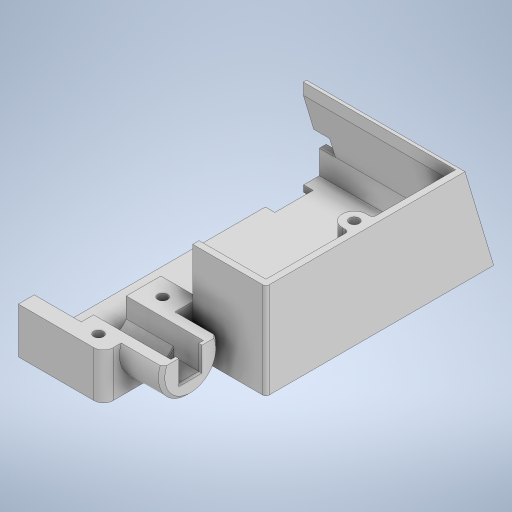
# Autodesk Inventor part: Tělo
Saved by Autodesk Inventor 2024 (Build 280153000, 153)
## iProperties
Created: 2023-04-15
Part Number: Tělo
Material: Všeobecné
Document SubType Name: Modeling
Designer: 42060
Density: 1 g/cm^3
Appearance: Výchozí
Author: 42060
Autodesk Inventor part; units mm, degrees
ref_plane "YZ Plane" through (0, 0, 0) normal (1, 0, 0) x (0, 1, 0)
ref_plane "XZ Plane" through (0, 0, 0) normal (0, 1, 0) x (-1, 0, 0)
ref_plane "XY Plane" through (0, 0, 0) normal (0, 0, 1) x (1, 0, 0)
sketch "Základ" plane through (0, 0, 0) normal (0, 0, 1) x (1, 0, 0)
  line L0 (0, 0) -> (49.75, 0)
  line L1 (49.75, 0) -> (49.75, -71.5)
  line L2 (49.75, -71.5) -> (26.75, -71.5)
  line L3 (26.75, -99.5) -> (0, -99.5)
  line L4 (0, -99.5) -> (0, 0)
  line L5 (0, -10) -> (47.75, -10)
  line L6 (47.75, -10) -> (47.75, -69.5)
  line L7 (47.75, -69.5) -> (14.75, -69.5)
  line L8 (14.75, -69.5) -> (14.75, -94.5)
  line L9 (14.75, -94.5) -> (0, -94.5)
  line L10 (26.75, -71.5) -> (26.75, -80.375)
  line L11 (26.75, -80.375) -> (26.75, -90.625)
  line L12 (26.75, -90.625) -> (26.75, -99.5)
  line L13 (26.75, -90.625) -> (14.75, -90.625)
  line L14 (26.75, -80.375) -> (14.75, -80.375)
  line L15 (26.75, -71.5) -> (26.75, -69.5)
  dimension "d0" = 49.75
  dimension "d1" = 99.5
  dimension "d3" = 2
  dimension "d5" = 28
  dimension "d14" = 10.25
  dimension "d15" = 12
  dimension "d16" = 5
  dimension "d17" = 23
  dimension "d18" = 2
  dimension "d19" = 10
  constraints: 32 end point, 8 perpendicular, 6 point on line, 3 horizontal, 2 collinear, 1 parallel, 1 vertical
  measures "d0" distance of L0.start L0.end
  measures "d1" distance between parallel lines of L3 L0
  measures "d3" distance between parallel lines of L1 L6
  measures "d5" distance of L2.end L3.start
  measures "d14" distance of L10.end L11.end
  measures "d15" distance between parallel lines of L8 L10
  measures "d16" distance between parallel lines of L9 L3
  measures "d17" distance between parallel lines of L1 L12
  measures "d18" distance between parallel lines of L2 L7
  measures "d19" distance between parallel lines of L0 L5
extrude "Podlaha" add sketch "Základ" along normal blind 2 contours L5 L6 L7 L8 L9 L4
extrude "Stěny" add sketch "Základ" along normal blind 30 contours L0 L1 L2 L15 L7 L6 L5 L4
extrude "Zadní stěny" add sketch "Základ" along normal blind 15 contours L9 L8 L13 L12 L3 L4 | L10 L14 L8 L7 L15
extrude "Stěna pod motorem" add sketch "Základ" along normal blind 5.25 contours L11 L13 L8 L14
sketch "Náčrt2" plane through (49.75, -71.5, 0) normal (1, 0, 0) x (0, 0, -1)
  line L0 (-2, 61.5) -> (-30, 61.5) projected
  line L1 (-2, 61.5) -> (-30, 61.5) projected
  line L2 (-30, 0) -> (-30, 71.5) projected
  line L3 (0, 71.5) -> (-30, 71.5) projected
  line L4 (0, 71.5) -> (0, 0) projected
  line L5 (-30, 62.5) -> (-10, 68.5)
  line L6 (-10, 68.5) -> (0, 71.5)
  dimension "d28" = 1
  dimension "d30" = 20
  constraints: 4 end point, 1 collinear, 1 point on line
  measures "d28" distance from line of L5.start L0
  measures "d30" horizontal distance of L5.end L5.start
extrude "Rampa" cut sketch "Náčrt2" against normal through all
sketch "Náčrt3" plane through (0, -10, 2) normal (-1, 0, 0) x (0, 0, 1)
  line L0 (0, 0) -> (28, 0) projected
  line L1 (0, 0) -> (28, 0) projected
  line L2 (24.3731, 0) -> (7.5, 5.0619)
  line L3 (7.5, 5.0619) -> (0, 5.0619)
  line L4 (0, 5.0619) -> (0, 0)
  line L5 (28, 1) -> (-2, 10) projected
  point P0 (-2, 10)
  point P1 (2, 7)
  point P2 (24.3731, 0)
  dimension "d34" = 7.5
  dimension "d37" = 2
  constraints: 6 end point, 1 horizontal, 1 perpendicular, 1 point on line, 2 other
  measures "d34" distance of L2.end L3.end
extrude "Přední rampa" cut sketch "Náčrt3" against normal up to surface (47.75 mm away)
sketch "Držák motoru" plane through (14.75, -94.5, 2) normal (-1, 0, 0) x (0, 0, 1)
  line L0 (3.25, 14.125) -> (13, 14.125) projected
  line L1 (3.25, 14.125) -> (3.25, 3.875) projected
  line L2 (3.25, 3.875) -> (13, 3.875) projected
  line L3 (6.13, 14.125) -> (12.37, 14.125)
  line L4 (12.37, 3.875) -> (6.13, 3.875)
  line L5 (3.25, 3.875) -> (13, 3.875) projected
  arc A0 (12.37, 3.875) -> (12.37, 14.125) centre (9.25, 9) ccw
  arc A1 (6.13, 14.125) -> (6.13, 3.875) centre (9.25, 9) ccw
  line L6 (15.25, 14.125) -> (15.25, 3.875) construction
  circle A2 centre (9.25, 9) radius 9
  line L7 (9.25, 18) -> (0, 18)
  line L8 (0, 0) -> (0, 89.5619) projected
  line L9 (0, 0) -> (13, 0) projected
  line L10 (13, -5) -> (13, 3.875) projected
  line L11 (0, 0) -> (13, 0) projected
  line L12 (0, 0) -> (13, 0) projected
  line L13 (12.37, 14.125) -> (12.37, 17.4419)
  line L14 (12.37, 3.875) -> (12.37, 0.5581)
  line L15 (12.37, 0.5581) -> (12.37, 0)
  line L16 (12.37, 17.4419) -> (12.37, 18)
  line L17 (12.37, 18) -> (9.25, 18)
  point P0 (-2, 94.5)
  point P1 (15.25, 9)
  point P2 (15.25, 9)
  point P3 (3.25, 9)
  point P4 (3.25, 9)
  point P5 (6.13, 3.875)
  point P6 (9.25, 0)
  point P7 (16.7333, 14)
  point P8 (16.7333, 4)
  point P9 (12.37, 0)
  dimension "d38" = 6
  dimension "d39" = 6
  dimension "d41" = 3
  dimension "d48" = 12
  constraints: 18 end point, 9 point on circle, 7 point on line, 4 tangent, 3 centre point, 3 coincident, 3 vertical, 2 horizontal alignment, 2 midpoint, 1 horizontal, 1 perpendicular
  measures "d38" radius of A0
  measures "d39" radius of A1
  measures "d41" radial gap between concentric circles of A2 A0
  measures "d48" distance between parallel lines of L1 L6
sketch "Náčrt10" plane through (14.75, -99.5, 0) normal (1, 0, 0) x (0, 0, -1)
  line L0 (-5.25, 8.875) -> (-15, 8.875) construction
  line L1 (-5.25, 8.875) -> (-17.25, 8.875) construction
  line L2 (-17.25, 8.875) -> (-17.25, 19.125) construction
  line L3 (-17.25, 19.125) -> (-5.25, 19.125) construction
  line L4 (-5.25, 19.125) -> (-5.25, 8.875) construction
  line L5 (-14.37, 8.875) -> (-8.13, 8.875)
  arc A0 (-8.13, 8.875) -> (-8.13, 19.125) centre (-11.25, 14) ccw
  line L6 (-14.37, 19.125) -> (-8.13, 19.125)
  arc A1 (-14.37, 5.5581) -> (-14.37, 22.4419) centre (-11.25, 14) ccw
  line L7 (-14.37, 8.875) -> (-14.37, 5.5581)
  line L8 (-14.37, 19.125) -> (-14.37, 22.4419)
  point P0 (0, 99.5)
  point P1 (-11.25, 19.125)
  point P2 (-11.25, 19.125)
  point P3 (-11.25, 8.875)
  point P4 (-11.25, 8.875)
  dimension "d79" = 12
  dimension "d80" = 6
  dimension "d81" = 18
  constraints: 16 end point, 5 point on line, 4 midpoint, 4 point on circle, 3 coincident, 2 centre point, 2 parallel, 2 perpendicular, 2 vertical alignment, 1 collinear, 1 horizontal, 1 horizontal alignment, 1 tangent
  measures "d79" distance between parallel lines of L4 L2
  measures "d80" radius of A0
  measures "d81" diameter of A1
extrude "Držák motoru (kulaté)" add sketch "Náčrt10" along normal blind 15
sketch "Náčrt11" plane through (29.75, -99.5, 0) normal (1, 0, 0) x (0, 0, -1)
  arc A0 (-8.13, 8.875) -> (-8.13, 19.125) centre (-11.25, 14) ccw projected
  circle A1 centre (-11.25, 14) radius 9
  line L0 (-17.25, 8.875) -> (-5.25, 8.875)
  line L1 (-5.25, 8.875) -> (-5.25, 19.125)
  line L2 (-5.25, 19.125) -> (-17.25, 19.125)
  line L3 (-17.25, 19.125) -> (-17.25, 8.875)
  line L4 (-17.25, 8.875) -> (-5.25, 19.125) construction
  line L5 (-5.25, 8.875) -> (-17.25, 19.125) construction
  line L6 (-14.37, 8.875) -> (-14.37, 5.5581) projected
  line L7 (-14.37, 22.4419) -> (-14.37, 19.125) projected
  point P0 (0, 99.5)
  dimension "d84" = 18
  constraints: 12 end point, 2 midpoint, 2 parallel, 1 centre point, 1 coincident, 1 horizontal, 1 horizontal alignment, 1 perpendicular, 1 tangent
  measures "d84" diameter of A1
extrude "Držák motoru (hranaté)" add sketch "Náčrt11" along normal blind 9.25 contours L0 L1 L2 L7 A1 L6
sketch "Spodní senzory" plane through (0, 0, 2) normal (0, 0, 1) x (1, 0, 0)
  line L0 (0, -4.9381) -> (47.75, -4.9381) projected
  line L1 (0, -94.5) -> (0, -4.9381) projected
  line L2 (0, -94.5) -> (14.75, -94.5) projected
  line L3 (14.75, -94.5) -> (14.75, -69.5) projected
  line L4 (14.75, -69.5) -> (47.75, -69.5) projected
  line L5 (47.75, -69.5) -> (47.75, -4.9381) projected
  line L6 (0, -24.4381) -> (5.5, -24.4381)
  line L7 (0, -21.9381) -> (3, -21.9381)
  line L8 (3, -21.9381) -> (3, -9.9381)
  line L9 (3, -9.9381) -> (0, -9.9381)
  line L10 (0, -7.4381) -> (5.5, -7.4381)
  line L11 (5.5, -7.4381) -> (5.5, -24.4381)
  line L12 (47.75, -22.8381) -> (36.75, -22.8381)
  line L13 (36.75, -22.8381) -> (36.75, -4.9381)
  line L14 (45.25, -20.3381) -> (39.25, -20.3381)
  line L15 (39.25, -20.3381) -> (39.25, -8.3381)
  line L16 (39.25, -8.3381) -> (45.25, -8.3381)
  line L17 (45.25, -8.3381) -> (45.25, -20.3381)
  point P0 (0, 0)
  dimension "d155" = 3
  dimension "d157" = 12
  dimension "d159" = 2.5
  dimension "d163" = 5
  dimension "d170" = 2.5
  dimension "d171" = 2.5
  dimension "d174" = 2.5
  dimension "d175" = 2.5
  dimension "d176" = 2.5
  dimension "d177" = 12
  dimension "d178" = 6
  dimension "d179" = 3.4
  constraints: 24 end point, 6 point on line, 5 perpendicular, 4 horizontal, 2 parallel, 1 vertical
  measures "d155" distance of L7.start L7.end
  measures "d157" distance of L7.end L8.end
  measures "d159" distance between parallel lines of L7 L6
  measures "d163" distance between parallel lines of L0 L9
  measures "d170" distance between parallel lines of L10 L9
  measures "d171" distance between parallel lines of L8 L11
  measures "d174" distance between parallel lines of L13 L15
  measures "d175" distance between parallel lines of L5 L17
  measures "d176" distance between parallel lines of L14 L12
  measures "d177" distance of L14.end L15.end
  measures "d178" distance of L14.start L14.end
  measures "d179" distance between parallel lines of L0 L16
extrude "Spodní senzory (díra)" cut sketch "Spodní senzory" against normal through all contours L9 L8 L7 L1 | L14 L15 L16 L17
extrude "Spodní senzory zvýšení" add sketch "Spodní senzory" along normal blind 10.5 contours L0 L5 L12 L13
sketch "Náčrt12" plane through (0, 0, 15) normal (0, 0, 1) x (1, 0, 0)
  line L0 (26.75, -80.375) -> (26.75, -71.5) projected
  line L1 (26.75, -69.5) -> (26.75, -71.5) projected
  line L2 (26.75, -69.5) -> (14.75, -69.5) projected
  line L3 (14.75, -69.5) -> (14.75, -80.375) projected
  line L4 (14.75, -80.375) -> (26.75, -80.375) projected
  line L5 (26.75, -99.5) -> (26.75, -90.625) projected
  line L6 (26.75, -90.625) -> (14.75, -90.625) projected
  line L7 (14.75, -90.625) -> (14.75, -94.5) projected
  line L8 (14.75, -94.5) -> (0, -94.5) projected
  line L9 (0, -94.5) -> (0, -99.5) projected
  line L10 (0, -99.5) -> (26.75, -99.5) projected
  point P0 (0, 0)
extrude "Vyrovnání držáku motoru" cut sketch "Náčrt12" against normal up to surface (0.63 mm away)
sketch "Náčrt13" plane through (14.75, -80.375, 14.37) normal (0, 0, 1) x (1, 0, 0)
  line L0 (0, 0) -> (0, 10.875) projected
  line L1 (0, 10.875) -> (12, 10.875) projected
  line L2 (0, -14.125) -> (0, -10.25) projected
  line L3 (0, -10.25) -> (24.25, -10.25) projected
  point P0 (-14.75, 80.375)
  point P1 (6, 5.4375)
  point P2 (6, -14.6875)
  dimension "d89" = 6
  dimension "d90" = 5.4375
  dimension "d91" = 6
  dimension "d92" = 4.4375
  measures "d89" distance from line of L0 point (6, 5.438)
  measures "d90" distance from line of L1 point (6, 5.438)
  measures "d91" distance from line of L2 point (6, -14.687)
  measures "d92" distance from line of L3 point (6, -14.687)
hole "Díry pro objímku motoru" at (20.75, -95.0625, 14.37) at (20.75, -74.9375, 14.37) direction (0, 0, -1) diameter 3 depth 6
fillet "Zaoblení stěny motoru" radius 3 1 edges at (26.75, -99.5, 7.185)
fillet "Zaoblení stěny" radius 1 1 edges at (49.75, -71.5, 15)
sketch "Náčrt14" plane through (39, -99.5, 0) normal (1, 0, 0) x (0, 0, -1)
  line L0 (-14.37, 19.125) -> (-5.25, 19.125) projected
  line L1 (-5.25, 19.125) -> (-5.25, 8.875) projected
  line L2 (-5.25, 8.875) -> (-14.37, 8.875) projected
  line L3 (-14.37, 8.875) -> (-14.37, 5.5581) projected
  arc A0 (-14.37, 5.5581) -> (-14.37, 22.4419) centre (-11.25, 14) ccw projected
  line L4 (-14.37, 22.4419) -> (-14.37, 19.125) projected
  line L5 (-14.37, 10.375) -> (-6.75, 10.375)
  line L6 (-6.75, 10.375) -> (-6.75, 17.625)
  line L7 (-6.75, 17.625) -> (-14.37, 17.625)
  line L8 (-14.37, 8.875) -> (-14.37, 10.375)
  line L9 (-14.37, 17.625) -> (-14.37, 19.125)
  point P0 (0, 99.5)
  dimension "d108" = 1.5
  dimension "d109" = 1.5
  dimension "d110" = 1.5
  constraints: 10 end point, 2 perpendicular, 2 point on line, 2 vertical, 2 vertical alignment
  measures "d108" distance between parallel lines of L5 L2
  measures "d109" distance between parallel lines of L1 L6
  measures "d110" distance between parallel lines of L0 L7
extrude "Vysunutí koncovky motoru" add sketch "Náčrt14" along normal blind 1
chamfer "Zkosení držáku motoru" distance 1 angle 45 1 edges at (40, -85.5, 2.25)
chamfer "Toleranční zkosení motoru" distance 0.25 angle 45 2 edges at (29.75, -88.4394, 6.0193) (29.75, -82.5606, 6.0193)
sketch "Náčrt16" plane through (0, 0, 30) normal (0, 0, 1) x (1, 0, 0)
  line L0 (47.75, -36) -> (45.75, -36)
  arc A0 (45.75, -36) -> (45.75, -43.5) centre (45.75, -39.75) ccw
  line L1 (45.75, -43.5) -> (47.75, -43.5)
  line L2 (47.75, -10) -> (47.75, -69.5) projected
  point P0 (47.75, -39.75)
  point P1 (47.75, -39.75)
  point P2 (47.75, -39.75)
  dimension "d130" = 3.75
  dimension "d131" = 2
  constraints: 4 end point, 3 midpoint, 2 coincident, 2 point on circle, 2 point on line, 2 tangent, 1 centre point, 1 horizontal, 1 horizontal alignment, 1 parallel
  measures "d130" radius of A0
  measures "d131" distance of L1.start L1.end
extrude "Vysunutí držáku PCB" add sketch "Náčrt16" against normal blind 10
sketch "Náčrt17" plane through (0, 0, 30) normal (0, 0, 1) x (1, 0, 0)
  arc A0 (45.75, -36) -> (45.75, -43.5) centre (45.75, -39.75) ccw projected
  point P0 (0, 0)
  constraints: 1 coincident
hole "Díra držáku PCB" at (45.75, -39.75, 30) direction (0, 0, -1) diameter 3 depth 6
sketch "Náčrt18" plane through (45.75, -43.5, 30) normal (0, -1, 0) x (1, 0, 0)
  line L0 (-10.625, -22) -> (-25.625, -22) projected
  line L1 (-3.75, -10) -> (0, -10) projected
  line L2 (0, -10) -> (2, -10) projected
  line L3 (-3.75, 0) -> (-3.75, -10) projected
  line L4 (-3.75, -6.6802) -> (2, -10)
  point P0 (-45.75, -30)
  dimension "d141" = 30
  constraints: 2 end point, 1 point on line
  measures "d141" angle of L1 L4
extrude "Zkosení PCB držáku" cut sketch "Náčrt18" against normal blind 10
fillet "Zaoblení hran" radius 1 11 edges at (46.75, -43.5, 20.5774) (46.75, -36, 20.5774) (43.0983, -42.4017, 22.6856) (43.0983, -37.0983, 22.6856) (47.75, -43.5, 25) (47.75, -36, 25) (47.75, -39.75, 20) (36.75, -22.8381, 7.25) (36.75, -4.9381, 5.75) (36.75, -5.3881, 11) (47.75, -22.8381, 7.25)
sketch "Náčrt22" plane through (0, -10, 30) normal (0, -1, 0) x (1, 0, 0)
  line L0 (0, -14.5) -> (5, -14.5)
  line L1 (5, -14.5) -> (5, -20.5)
  line L2 (5, -20.5) -> (0, -20.5)
  line L3 (0, -20.5) -> (0, -14.5)
  line L4 (0, -28) -> (35.75, -28) projected
  line L5 (0, -20.5) -> (0, -3.6269) projected
  point P0 (0, -30)
  point P1 (36.75, -28)
  dimension "d180" = 7.5
  dimension "d181" = 6
  dimension "d182" = 5
  constraints: 8 end point, 2 parallel, 1 collinear, 1 horizontal, 1 perpendicular
  measures "d180" distance between parallel lines of L2 L4
  measures "d181" distance of L0.end L1.end
  measures "d182" distance of L1.end L2.end
extrude "Přední senzor" cut sketch "Náčrt22" against normal through all
sketch "Náčrt15" plane through (49.75, -70.5, 0) normal (1, 0, 0) x (0, 0, -1)
  line L0 (-20.5, 9) -> (-20.5, 54) construction
  line L1 (-20.5, 54) -> (-9.5, 54) construction
  line L2 (-9.5, 54) -> (-9.5, 9) construction
  line L3 (-9.5, 9) -> (-20.5, 9) construction
  line L4 (-30, -1) -> (0, -1) projected
  line L5 (0, 0) -> (0, 70.5) projected
  point P0 (-15, 9)
  point P1 (-15, -1)
  point P2 (-9.5, 31.5)
  point P3 (0, 35.25)
  dimension "d145" = 11
  dimension "d146" = 45
  dimension "d185" = 10
  constraints: 4 midpoint, 1 vertical alignment, 2 other
  measures "d145" distance of L0.end L1.end
  measures "d146" distance of L1.end L2.end
  measures "d185" distance between parallel lines of L4 L3
sketch "Náčrt19" plane through (-49.75, -70.5, 0) normal (-1, 0, 0) x (0, 0, 1)
  line L0 (20.5, 54) -> (20.5, 9) construction
  line L1 (20.5, 9) -> (9.5, 9) construction
  line L2 (9.5, 9) -> (9.5, 54) construction
  line L3 (9.5, 54) -> (20.5, 54) construction
  line L4 (30, -1) -> (0, -1) projected
  line L5 (0, 0) -> (0, 70.5) projected
  point P0 (15, 9)
  point P1 (15, -1)
  point P2 (9.5, 31.5)
  point P3 (0, 35.25)
  dimension "d149" = 11
  dimension "d150" = 45
  dimension "d186" = 10
  constraints: 4 midpoint, 1 vertical alignment, 2 other
  measures "d149" distance of L0.end L1.end
  measures "d150" distance of L1.end L2.end
  measures "d186" distance between parallel lines of L4 L1
